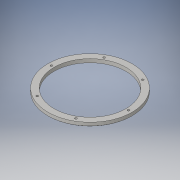
# Autodesk Inventor part: Oring Fitting Dome V2 -part
Saved by Autodesk Inventor 2016 (Build 200138000, 138)
## iProperties
Created: 2017-03-08
Part Number: Oring Fitting Dome V2 -part
Material: Generic
Document SubType Name: Modeling
Designer: Student
Density: 1 g/cm^3
Appearance: Default
Author: Student
Autodesk Inventor part; units mm, degrees
ref_plane "YZ Plane" through (0, 0, 0) normal (1, 0, 0) x (0, 1, 0)
ref_plane "XZ Plane" through (0, 0, 0) normal (0, 1, 0) x (-1, 0, 0)
ref_plane "XY Plane" through (0, 0, 0) normal (0, 0, 1) x (1, 0, 0)
sketch "Sketch1" plane through (0, 0, 0) normal (0, 1, 0) x (-1, 0, 0)
  circle A0 centre (0, 0) radius 51.435
  circle A1 centre (0, 0) radius 60.198
  dimension "d0" = 102.87
  dimension "d1" = 120.396
  constraints: 2 centre point, 2 coincident
  measures "d0" diameter of A0
  measures "d1" diameter of A1
extrude "Extrusion1" add sketch "Sketch1" along normal blind 5.08
sketch "Sketch2" plane through (0, 5.08, 0) normal (0, 1, 0) x (1, 0, 0)
  circle A0 centre (0, 0) radius 55.245
  point P0 (-55.245, 0)
  point P1 (-27.6225, -47.8436)
  point P2 (27.6225, -47.8436)
  point P3 (55.245, 0)
  point P4 (27.6225, 47.8436)
  point P5 (-27.6225, 47.8436)
  dimension "d4" = 110.49
  dimension "d8" = 360
  constraints: 1 coincident, 1 horizontal alignment, 9 other
hole "Hole1" at (-55.245, 5.08, 0) at (-27.6225, 5.08, 47.8436) at (27.6225, 5.08, 47.8436) at (55.245, 5.08, 0) at (27.6225, 5.08, -47.8436) at (-27.6225, 5.08, -47.8436) direction (0, -1, 0) diameter 3 end through all
chamfer "Chamfer1" distance 0.508 angle 45 1 edges at (60.198, 0, 0)
body "Solid1"
